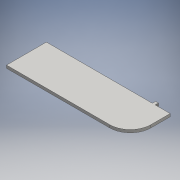
# Autodesk Inventor part: boxgeneric
Saved by Autodesk Inventor 2016 (Build 200138000, 138)
## iProperties
Created: 2015-12-29
Part Number: boxgeneric
Material: Generic
Document SubType Name: Modeling
Designer: hesaon
Density: 1 g/cm^3
Appearance: Default
Author: hesaon
Autodesk Inventor part; units mm, degrees
ref_plane "YZ Plane" through (0, 0, 0) normal (1, 0, 0) x (0, 1, 0)
ref_plane "XZ Plane" through (0, 0, 0) normal (0, 1, 0) x (-1, 0, 0)
ref_plane "XY Plane" through (0, 0, 0) normal (0, 0, 1) x (1, 0, 0)
sketch "Sketch1" plane through (0, 0, 0) normal (0, 0, 1) x (1, 0, 0)
  line L0 (0, 0) -> (110, 0)
  line L1 (0, 42.5) -> (0, 0)
  line L2 (132, 42.5) -> (116, 42.5)
  line L3 (116, 42.5) -> (116, 46)
  line L4 (116, 46) -> (113, 46)
  line L5 (113, 46) -> (113, 42.5)
  line L6 (113, 42.5) -> (110, 42.5)
  arc A0 (110, 0) -> (132, 22) centre (110, 22) ccw
  line L7 (110, 22) -> (110, 0) construction
  line L8 (132, 22) -> (132, 42.5)
  line L9 (132, 42.5) -> (116, 42.5)
  line L10 (113, 42.5) -> (0, 42.5)
  dimension "d2" = 16
  dimension "d3" = 3.5
  dimension "thickness" = 3
  dimension "d5" = 3
  dimension "d14" = 110
  dimension "d15" = 22
  dimension "d16" = 22
  dimension "d17" = 20.5
  dimension "d18" = 110
  dimension "d19" = 90
  dimension "d20" = 3
  constraints: 22 end point, 6 perpendicular, 2 point on circle, 1 centre point, 1 horizontal, 1 point on line, 1 vertical
  measures "d2" distance of L2.start L2.end
  measures "d3" distance of L2.end L3.end
  measures "thickness" distance of L3.end L4.end
  measures "d5" distance of L5.end L6.end
  measures "d14" distance of L0.start L0.end
  measures "d15" distance of L7.start L8.start
  measures "d16" horizontal distance of L8.start L0.end
  measures "d17" distance of L8.start L2.start
  measures "d18" distance of L6.end L1.start
  measures "d20" distance of L2.end L5.end
extrude "Extrusion1" add sketch "Sketch1" along normal blind 3
equation "\"d5\" = thickness"
equation "\"d20\" = thickness"
equation "\"d21\" = thickness"
body "Solid1"
